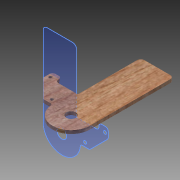
# Autodesk Inventor part: p6
Saved by Autodesk Inventor 2015 (Build 190159000, 159)
## iProperties
Created: 2016-02-03
Part Number: p6
Material: Generic
Document SubType Name: Modeling
Designer: david
Density: 1 g/cm^3
Appearance: Birch - Natural Polished
Mass: 6.40214 g
Surface Area: 43.8659 cm^2
Volume: 6.40214 cm^3
Author: david
Autodesk Inventor part; units mm, degrees
ref_plane "YZ Plane" through (0, 0, 0) normal (1, 0, 0) x (0, 1, 0)
ref_plane "XZ Plane" through (0, 0, 0) normal (0, 1, 0) x (-1, 0, 0)
ref_plane "XY Plane" through (0, 0, 0) normal (0, 0, 1) x (1, 0, 0)
sketch "Sketch1" plane through (0, 0, 0) normal (0, 0, 1) x (1, 0, 0)
  circle A0 centre (25.0558, -45.1154) radius 20
  line L0 (45.0558, -45.1154) -> (31.0558, -45.1154)
  line L1 (31.0558, -45.1154) -> (31.0558, -22.1154)
  line L2 (31.0558, -22.1154) -> (45.0558, -22.1154)
  line L3 (45.0558, -22.1154) -> (45.0558, -45.1154)
  line L4 (31.0558, -22.1154) -> (-4.9442, -22.1154)
  line L5 (-4.9442, -22.1154) -> (-4.9442, -45.1154)
  line L6 (-4.9442, -45.1154) -> (31.0558, -45.1154)
  line L7 (31.0558, -45.1154) -> (31.0558, -22.1154)
  line L8 (-4.9442, -45.1154) -> (-24.9442, -25.1154)
  line L9 (-24.9442, -25.1154) -> (-24.9442, -15.1154)
  line L10 (-24.9442, -15.1154) -> (-4.9442, -15.1154)
  line L11 (-4.9442, -15.1154) -> (-4.9442, -22.1154)
  point P0 (0, 0)
  dimension "d0" = 40
  dimension "d1" = 14
  dimension "d2" = 23
  dimension "d20" = 0
  dimension "d21" = 23
  dimension "d22" = 30
  dimension "d23" = 20
  dimension "d24" = 50
  dimension "d45" = 10
  constraints: 24 end point, 4 parallel, 4 perpendicular, 2 horizontal, 1 horizontal alignment, 1 point on line, 1 vertical, 2 other
  measures "d1" distance of L1.end L2.end
  measures "d2" distance of L0.end L1.end
  measures "d20" distance between parallel lines of L2 L4
  measures "d21" distance between parallel lines of L4 L6
  measures "d22" distance from line of L10 L5.end
  measures "d23" distance between parallel lines of L11 L9
  measures "d24" distance between parallel lines of L3 L5
  measures "d45" distance of L8.end L9.end
extrude "Extrusion1" add sketch "Sketch1" along normal blind 3.6
sketch "Sketch2" plane through (0, 0, 3.6) normal (0, 0, 1) x (1, 0, 0)
  arc A0 (5.0558, -45.1154) -> (45.0558, -45.1154) centre (25.0558, -45.1154) ccw projected
  circle A1 centre (25.0558, -45.1154) radius 5.15
  circle A2 centre (0.0558, -40.8364) radius 1.625
  line L0 (-4.9442, -22.1154) -> (-4.9442, -45.1154) projected
  line L1 (-4.9442, -45.1154) -> (5.0558, -45.1154) projected
  line L2 (45.0558, -45.1154) -> (45.0558, -22.1154) projected
  line L3 (45.0558, -22.1154) -> (-4.9442, -22.1154) projected
  circle A3 centre (-21.4442, -20.8364) radius 1.625
  point P0 (0, 0)
  point P1 (30.9974, -15.1154)
  dimension "d5" = 10.3
  dimension "d6" = 3.25
  dimension "d10" = 4.279
  dimension "d18" = 23
  dimension "d25" = 3.25
  dimension "d26" = 20
  dimension "d27" = 21.5
  constraints: 3 centre point, 1 coincident, 1 other
  measures "d5" diameter of A1
  measures "d6" diameter of A2
  measures "d10" distance from line of L1 A2.centre
  measures "d25" diameter of A3
  measures "d26" vertical distance of A2.centre A3.centre
  measures "d27" horizontal distance of A3.centre A2.centre
extrude "Extrusion2" cut sketch "Sketch2" against normal blind 20 contours A1 | A2 | A3
fillet "Fillet1" radius 2 3 edges at (45.0558, -22.1154, 1.8) (-4.9442, -45.1154, 1.8) (5.0558, -45.1154, 1.8)
fillet "Fillet2" radius 3 4 edges at (-24.9442, -25.1154, 1.8) (-24.9442, -15.1154, 1.8) (-4.9442, -15.1154, 1.8) (-4.9442, -22.1154, 1.8)
sketch "Sketch3" plane through (0, 0, 0) normal (0, 0, -1) x (-1, 0, 0)
  line L0 (7.9442, -15.1154) -> (21.9442, -15.1154) projected
  line L1 (14.9442, -15.1154) -> (-0.0558, -15.1154)
  line L2 (-0.0558, -15.1154) -> (-0.0558, -22.1154)
  line L3 (-0.0558, -22.1154) -> (14.9442, -22.1154)
  line L4 (14.9442, -22.1154) -> (14.9442, -15.1154)
  line L5 (4.9442, -19.1154) -> (4.9442, -18.1154) projected
  point P0 (0, 0)
  dimension "d29" = 7
  dimension "d32" = 15
  dimension "d33" = 5
  constraints: 8 end point, 2 parallel, 1 horizontal, 1 midpoint, 1 perpendicular
  measures "d29" distance between parallel lines of L1 L3
  measures "d32" distance of L2.end L3.end
  measures "d33" distance between parallel lines of L5 L2
extrude "Extrusion3" cut sketch "Sketch3" against normal blind 10
fillet "Fillet3" radius 3 2 edges at (-14.9442, -15.1154, 1.8) (-14.9442, -22.1154, 1.8)
sketch "Sketch4" plane through (0, 0, 0) normal (0, 0, -1) x (-1, 0, 0)
  line L0 (-45.0558, -45.1154) -> (-45.0558, -24.1154) projected
  line L1 (-45.0558, -28.8196) -> (-9.3289, -28.8196)
  line L2 (-9.3289, -28.8196) -> (-9.3289, 45.6636)
  line L3 (-9.3289, 45.6636) -> (-45.0558, 45.6636)
  line L4 (-45.0558, 45.6636) -> (-45.0558, -28.8196)
  line L5 (-43.0558, -22.1154) -> (11.9442, -22.1154) projected
  circle A0 centre (-0.0558, -40.8364) radius 1.625 projected
  point P0 (0, 0)
  dimension "d36" = 86.5
  constraints: 8 end point, 2 parallel, 1 horizontal, 1 perpendicular, 1 point on line
  measures "d36" distance from line of L3 A0.centre
extrude "Extrusion4" add sketch "Sketch4" against normal blind 3.6 contours L0 L4 L3 L2 L1
fillet "Fillet4" radius 4 2 edges at (9.3289, 45.6636, 1.8) (45.0558, 45.6636, 1.8)
sketch "Sketch5" plane through (0, 0, 0) normal (0, 0, -1) x (-1, 0, 0)
  circle A0 centre (-41.5558, 42.1636) radius 1.625
  line L0 (-13.3289, 45.6636) -> (-41.0558, 45.6636) projected
  line L1 (-45.0558, 41.6636) -> (-45.0558, -45.1154) projected
  point P0 (0, 0)
  point P1 (-41.0558, 41.6636)
  dimension "d40" = 3.25
  dimension "d43" = 3.5
  dimension "d44" = 3.5
  constraints: 1 centre point
  measures "d40" diameter of A0
  measures "d43" distance from line of L0 A0.centre
  measures "d44" distance from line of L1 A0.centre
extrude "Extrusion5" cut sketch "Sketch5" against normal blind 3
body "Solid1"
